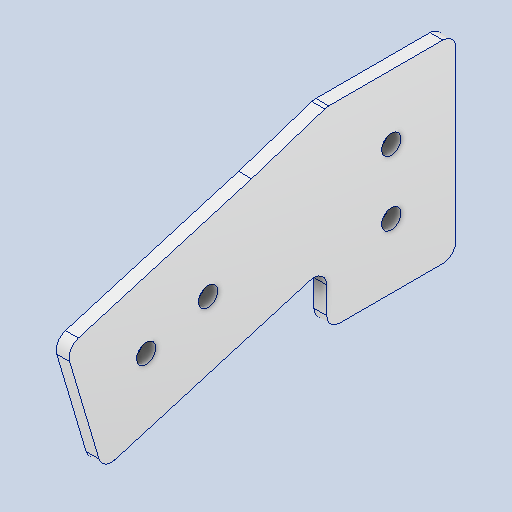
# Autodesk Inventor part: dribl-v1-Plate-10
Saved by Autodesk Inventor 2025.2 (Build 292293000, 293)
## iProperties
Created: 2025-01-13
Part Number: dribl-v1-Plate-10
Material: アルミニウム 6061
Document SubType Name: Modeling
Designer: haruy
Density: 2.7 g/cm^3
Appearance: アルミニウム - フラット
Author: haruy
Autodesk Inventor part; units mm, degrees
ref_plane "YZ Plane" through (0, 0, 0) normal (1, 0, 0) x (0, 1, 0)
ref_plane "XZ Plane" through (0, 0, 0) normal (0, 1, 0) x (-1, 0, 0)
ref_plane "XY Plane" through (0, 0, 0) normal (0, 0, 1) x (1, 0, 0)
sketch "スケッチ1" plane through (0, 0, 0) normal (1, 0, 0) x (0, 1, 0)
  line L0 (-64.254, -635.7138) -> (-64.254, 672.2862)
  line L1 (-64.254, -533.7138) -> (340.746, -533.7138)
  line L2 (340.746, -533.7138) -> (340.746, -513.7138)
  line L3 (340.746, -513.7138) -> (-64.254, -513.7138)
  line L4 (-64.254, -513.7138) -> (-64.254, -533.7138)
  circle A0 centre (-29.074, -486.7138) radius 21
  circle A1 centre (-29.074, -444.7138) radius 16
  circle A2 centre (-29.074, -444.7138) radius 13.68
  line L5 (-84.254, -635.7138) -> (-64.254, -635.7138)
  line L6 (-84.254, -635.7138) -> (-64.254, -635.7138)
  line L7 (-84.254, -635.7138) -> (399.746, -635.7138)
  line L8 (399.746, -635.7138) -> (399.746, -655.7138)
  line L9 (399.746, -655.7138) -> (-84.254, -655.7138)
  line L10 (-84.254, -655.7138) -> (-84.254, -635.7138)
  line L11 (-9.074, 672.2862) -> (10.1017, 677.9687)
  line L12 (10.1017, 677.9687) -> (395.949, -624.0627)
  line L13 (395.949, -624.0627) -> (376.7733, -629.7453)
  line L14 (376.7733, -629.7453) -> (-9.074, 672.2862)
  line L15 (-84.254, 672.2862) -> (-84.254, -635.7138)
  line L16 (-84.254, -428.7138) -> (-29.074, -428.7138)
  line L17 (-8.074, -486.7138) -> (-8.074, -533.7138)
  line L18 (-8.074, -486.7138) -> (-8.074, -428.7138)
  line L19 (-8.074, -428.7138) -> (-29.074, -428.7138)
  circle A3 centre (-74.254, -440.7138) radius 1.5
  circle A4 centre (-74.254, -450.7138) radius 1.5
  line L20 (-29.074, -460.7138) -> (-84.254, -460.7138)
  circle A5 centre (-54.254, -523.7138) radius 1.5
  circle A6 centre (-34.254, -523.7138) radius 1.5
  line L21 (-64.254, -533.7138) -> (-84.254, -533.7138)
  circle A7 centre (-74.254, -523.7138) radius 1.5
  circle A8 centre (-74.254, -503.7138) radius 1.5
  circle A9 centre (-29.074, 656.2862) radius 16
  line L22 (-64.254, 672.2862) -> (-84.254, 672.2862)
  line L23 (-84.254, 672.2862) -> (-29.074, 672.2862)
  line L24 (-29.074, 640.2862) -> (-84.254, 640.2862)
  line L25 (-29.074, 672.2862) -> (-9.074, 672.2862)
  circle A10 centre (-29.074, 656.2862) radius 7.5
  line L26 (-29.074, 640.2862) -> (0.4089, 640.2862)
  circle A11 centre (-74.254, 660.2862) radius 1.5
  circle A12 centre (-74.254, 650.2862) radius 1.5
  circle A13 centre (3.3551, 665.5396) radius 1.5
  circle A14 centre (6.1964, 655.9517) radius 1.5
  line L27 (0.4089, 640.2862) -> (19.5847, 645.9687)
  line L28 (-64.254, -595.7138) -> (-44.254, -635.7138)
  line L29 (-44.254, -635.7138) -> (-44.254, -655.7138)
  line L30 (-64.254, -595.7138) -> (-84.254, -595.7138)
  circle A15 centre (-74.254, -625.7138) radius 1.5
  circle A16 centre (-74.254, -615.7138) radius 1.5
  circle A17 centre (-74.254, -605.7138) radius 1.5
  circle A18 centre (-74.254, -645.7138) radius 1.5
  circle A19 centre (-64.254, -645.7138) radius 1.5
  circle A20 centre (-54.254, -645.7138) radius 1.5
  line L31 (-84.254, -635.7138) -> (-84.254, -595.7138)
  line L32 (369.746, -635.7138) -> (369.746, -655.7138)
  line L33 (368.2494, -600.9817) -> (387.4252, -595.2991)
  line L34 (376.7733, -629.7453) -> (378.5421, -635.7138)
  line L35 (395.949, -624.0627) -> (399.746, -635.7138)
  circle A21 centre (379.746, -645.7138) radius 1.5
  circle A22 centre (389.746, -645.7138) radius 1.5
  circle A23 centre (383.5199, -617.3161) radius 1.5
  circle A24 centre (380.6786, -607.7283) radius 1.5
  circle A25 centre (320.746, -523.7138) radius 1.5
  circle A26 centre (330.746, -523.7138) radius 1.5
  line L36 (340.746, -513.7138) -> (342.3883, -513.7138)
  line L37 (340.746, -533.7138) -> (348.3151, -533.7138)
  line L38 (342.3883, -513.7138) -> (363.248, -513.7138)
  circle A27 centre (355.6752, -523.3551) radius 1.5
  circle A28 centre (358.5165, -532.9429) radius 1.5
  line L39 (351.7699, -545.3721) -> (370.9457, -539.6895)
  line L40 (310.746, -513.7138) -> (310.746, -533.7138)
  line L41 (368.2494, -600.9817) -> (369.746, -635.7138)
  point P0 (0, 0)
  point P1 (-387.254, -203.3804)
  point P2 (-64.254, -513.7138)
  point P3 (386.3612, -626.904)
  dimension "d1" = 42
  dimension "d0" = 20
  dimension "d2" = 32
  dimension "d3" = 27.36
  dimension "d4" = 35.18
  dimension "d5" = 35.18
  dimension "d6" = 27
  dimension "d7" = 42
  dimension "d8" = 191
  dimension "d9" = 20
  dimension "d10" = 484
  dimension "d11" = 3
  dimension "d12" = 3
  dimension "d13" = 10
  dimension "d14" = 10
  dimension "d15" = 10
  dimension "d16" = 10
  dimension "d17" = 3
  dimension "d18" = 3
  dimension "d19" = 10
  dimension "d20" = 20
  dimension "d21" = 10
  dimension "d22" = 10
  dimension "d23" = 3
  dimension "d24" = 3
  dimension "d25" = 10
  dimension "d26" = 20
  dimension "d27" = 10
  dimension "d28" = 10
  dimension "d29" = 20
  dimension "d30" = 32
  dimension "d31" = 35.18
  dimension "d32" = 20
  dimension "d33" = 1358
  dimension "d34" = 91.543
  dimension "d35" = 405
  dimension "d36" = 15
  dimension "d37" = 3
  dimension "d38" = 3
  dimension "d39" = 10
  dimension "d40" = 10
  dimension "d41" = 10
  dimension "d42" = 10
  dimension "d43" = 3
  dimension "d44" = 3
  dimension "d45" = 10
  dimension "d46" = 10
  dimension "d47" = 10
  dimension "d48" = 10
  dimension "d49" = 40
  dimension "d50" = 3
  dimension "d51" = 3
  dimension "d52" = 3
  dimension "d53" = 3
  dimension "d54" = 3
  dimension "d55" = 3
  dimension "d56" = 10
  dimension "d57" = 10
  dimension "d58" = 10
  dimension "d59" = 10
  dimension "d60" = 10
  dimension "d61" = 10
  dimension "d62" = 10
  dimension "d63" = 10
  dimension "d64" = 10
  constraints: 84 end point, 28 centre point, 28 point on line, 14 perpendicular, 7 parallel, 7 tangent, 5 point on circle, 3 horizontal, 3 vertical, 2 coincident, 2 collinear, 1 horizontal alignment, 1 midpoint, 2 other
  measures "d0" distance of L2.end L1.end
  measures "d2" diameter of A1
  measures "d3" diameter of A2
  measures "d4" distance from line of L0 A1.centre
  measures "d5" distance from line of point (-29.074, -486.714) L0
  measures "d6" distance from line of L3 point (-29.074, -486.714)
  measures "d7" distance of point (-29.074, -486.714) A1.centre
  measures "d8" distance from line of A1.centre L5
  measures "d9" distance of L7.end L8.end
  measures "d10" distance between parallel lines of L10 L8
  measures "d11" diameter of A3
  measures "d12" diameter of A4
  measures "d13" distance of A4.centre A3.centre
  measures "d14" distance from line of A3.centre L0
  measures "d15" distance from line of A4.centre L20
  measures "d16" distance from line of L0 A4.centre
  measures "d17" diameter of A5
  measures "d18" diameter of A6
  measures "d19" distance from line of A5.centre L0
  measures "d20" distance of A6.centre A5.centre
  measures "d21" distance from line of A5.centre L1
  measures "d22" distance from line of A6.centre L1
  measures "d23" diameter of A7
  measures "d24" diameter of A8
  measures "d25" distance from line of A7.centre L21
  measures "d26" distance of A8.centre A7.centre
  measures "d27" distance from line of A8.centre L15
  measures "d28" distance from line of L15 A7.centre
  measures "d29" distance between parallel lines of L14 L12
  measures "d30" diameter of A9
  measures "d31" distance from line of L0 A9.centre
  measures "d32" horizontal distance of L11.start A9.centre
  measures "d33" distance between parallel lines of L11 L13
  measures "d35" distance between parallel lines of L0 L2
  measures "d36" diameter of A10
  measures "d37" diameter of A11
  measures "d38" diameter of A12
  measures "d39" distance from line of A12.centre L24
  measures "d40" distance of A11.centre A12.centre
  measures "d41" distance from line of A12.centre L0
  measures "d42" distance from line of A11.centre L0
  measures "d43" diameter of A13
  measures "d44" diameter of A14
  measures "d45" distance from line of A13.centre L11
  measures "d46" distance from line of A13.centre L12
  measures "d47" distance of A13.centre A14.centre
  measures "d48" distance from line of A14.centre L12
  measures "d49" distance between parallel lines of L10 L29
  measures "d50" diameter of A15
  measures "d51" diameter of A16
  measures "d52" diameter of A17
  measures "d53" diameter of A18
  measures "d54" diameter of A19
  measures "d55" diameter of A20
  measures "d56" distance from line of A18.centre L9
  measures "d57" distance from line of A18.centre L10
  measures "d58" distance of A19.centre A18.centre
  measures "d59" distance from line of A19.centre L9
  measures "d60" distance from line of A20.centre L9
  measures "d61" distance of A19.centre A20.centre
  measures "d62" distance from line of A15.centre L7
  measures "d63" distance from line of A15.centre L0
  measures "d64" distance of A16.centre A15.centre
extrude "押し出し1" add sketch "スケッチ1" against normal blind 2 contours L7 L8 L9 L32 | L34 L13 L35 L7 | L33 L12 L13 L14
fillet "フィレット1" radius 2 7 edges at (-1, 368.2494, -600.9817) (-1, 378.5421, -635.7138) (-1, 369.746, -635.7138) (-1, 369.746, -655.7138) (-1, 399.746, -655.7138) (-1, 399.746, -635.7138) (-1, 387.4252, -595.2991)
equation "\"d5\" = d4"
equation "\"d14\" = d15"
equation "\"d21\" = d19"
equation "\"d22\" = d19"
equation "\"d27\" = d25"
equation "\"d28\" = d25"
equation "\"d31\" = d4"
equation "\"d41\" = d39"
equation "\"d42\" = d39"
equation "\"d46\" = d45"
equation "\"d47\" = d45"
equation "\"d48\" = d45"
equation "\"d57\" = d56"
equation "\"d58\" = d56"
equation "\"d59\" = d56"
equation "\"d60\" = d56"
equation "\"d61\" = d56"
equation "\"d62\" = d56"
equation "\"d63\" = d56"
equation "\"d64\" = d62"
